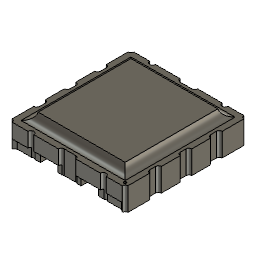
MGF0918A (Autodesk Fusion 360 design; units mm, degrees)
part number: 2026-08-04-15-31-29-317
Autodesk Fusion 360 part; units mm, degrees
sketch "Sketch1" plane through (0, 0, 0) normal (0, 0, 1) x (1, 0, 0)
  line L0 (2, 2.1) -> (-2, 2.1)
  line L1 (-2, 2.1) -> (-2, -2.1)
  line L2 (-2, -2.1) -> (2, -2.1)
  line L3 (2, -2.1) -> (2, 2.1)
  line L4 (2, 2.1) -> (-2, -2.1) construction
  line L5 (-2, 2.1) -> (2, -2.1) construction
  dimension "d1" = 4
  dimension "d2" = 4.2
  constraint horizontal L0
  constraint perpendicular L0 L1
  constraint parallel L0 L2
  constraint parallel L1 L3
  constraint coincident L4 origin
  constraint coincident L5 origin
  measures "d1" distance of L1.end L2.end
  measures "d2" distance of L0.end L1.end
extrude "Extrude1" add sketch "Sketch1" along normal blind 0.8
sketch "Sketch2" plane through (0, 0, 0.8) normal (0, 0, 1) x (-1, 0, 0)
  line L0 (-2, 2.1) -> (-2, -2.1)
  line L1 (-2, -2.1) -> (2, -2.1)
  line L2 (2, -2.1) -> (2, 2.1)
  line L3 (2, 2.1) -> (-2, 2.1)
sketch "Sketch3" plane through (0, 0, 0.8) normal (0, 0, 1) x (-1, 0, 0)
  line L0 (-2, -2.1) -> (2, -2.1)
  line L1 (-1.5, -1.6) -> (1.5, -1.6)
  line L2 (1.5, -1.6) -> (1.5, 1.6)
  line L3 (1.5, 1.6) -> (-1.5, 1.6)
  line L4 (-1.5, 1.6) -> (-1.5, -1.6)
  line L5 (-1.5, -1.6) -> (1.5, 1.6) construction
  line L6 (1.5, -1.6) -> (-1.5, 1.6) construction
  dimension "d5" = 4
  dimension "d6" = 3
  dimension "d7" = 3.2
  constraint horizontal L1
  constraint perpendicular L1 L2
  constraint parallel L1 L3
  constraint parallel L2 L4
  constraint coincident L5 origin
  constraint coincident L6 origin
  measures "d5" distance of L0.start L0.end
  measures "d6" distance of L2.end L3.end
  measures "d7" distance of L1.end L2.end
extrude "Extrude2" add sketch "Sketch3" along normal blind 0.25
sketch "Sketch4" plane through (0, 0, 0) normal (0, 0, -1) x (1, 0, 0)
  line L0 (2, -2.1) -> (2, 2.1)
  line L1 (2, 2.1) -> (-2, 2.1)
  line L2 (-2, 2.1) -> (-2, -2.1)
  line L3 (-2, -2.1) -> (2, -2.1)
  line L4 (-2, -2.1) -> (2, -2.1) construction
  line L5 (0, -2.1) -> (0, -2) construction
  line L6 (0.3, -2.1) -> (0.3, -2) construction
  line L7 (-0.3, -2.1) -> (-0.3, -2) construction
  line L8 (1.25, -2.1) -> (1.25, -2) construction
  line L9 (-1.25, -2.1) -> (-1.25, -2) construction
  line L10 (1.35, -2.1) -> (1.35, -2) construction
  line L11 (1.15, -2.1) -> (1.15, -2) construction
  line L12 (1.35, -2.1) -> (1.15, -2.1)
  arc A0 (1.25, -2) -> (1.15, -2.1) centre (1.25, -2.1) ccw
  arc A1 (1.35, -2.1) -> (1.25, -2) centre (1.25, -2.1) ccw
  arc A2 (-1.25, -2) -> (-1.35, -2.1) centre (-1.25, -2.1) ccw
  arc A3 (-1.15, -2.1) -> (-1.25, -2) centre (-1.25, -2.1) ccw
  line L13 (-1.15, -2.1) -> (-1.35, -2.1)
  line L14 (-0.2, -2) -> (0.2, -2)
  line L15 (0.3, -2.1) -> (-0.3, -2.1)
  arc A4 (-0.2, -2) -> (-0.3, -2.1) centre (-0.2, -2.1) ccw
  arc A5 (0.3, -2.1) -> (0.2, -2) centre (0.2, -2.1) ccw
  arc A6 (1.15, 2.1) -> (1.25, 2) centre (1.25, 2.1) ccw
  arc A7 (1.25, 2) -> (1.35, 2.1) centre (1.25, 2.1) ccw
  line L16 (-0.2, 2) -> (0.2, 2)
  arc A8 (-0.3, 2.1) -> (-0.2, 2) centre (-0.2, 2.1) ccw
  arc A9 (0.2, 2) -> (0.3, 2.1) centre (0.2, 2.1) ccw
  arc A10 (-1.35, 2.1) -> (-1.25, 2) centre (-1.25, 2.1) ccw
  arc A11 (-1.25, 2) -> (-1.15, 2.1) centre (-1.25, 2.1) ccw
  line L17 (1.35, 2.1) -> (1.15, 2.1)
  line L18 (-0.3, 2.1) -> (0.3, 2.1)
  line L19 (-1.15, 2.1) -> (-1.35, 2.1)
  line L20 (0, 0) -> (2, 0) construction
  line L21 (0, 0) -> (-2, 0) construction
  line L22 (2, 0) -> (2, 0.2)
  line L23 (2, 0) -> (2, -0.2)
  line L24 (1.9, 0.1) -> (1.9, -0.1)
  arc A12 (2, 0.2) -> (1.9, 0.1) centre (2, 0.1) ccw
  arc A13 (1.9, -0.1) -> (2, -0.2) centre (2, -0.1) ccw
  arc A14 (-2, -0.2) -> (-1.9, -0.1) centre (-2, -0.1) ccw
  line L25 (-2, 0) -> (-2, -0.2)
  line L26 (-2, 0) -> (-2, 0.2)
  arc A15 (-1.9, 0.1) -> (-2, 0.2) centre (-2, 0.1) ccw
  line L27 (-1.9, 0.1) -> (-1.9, -0.1)
  arc A16 (1.9, 0.95) -> (2, 0.85) centre (2, 0.95) ccw
  line L28 (2, 1.05) -> (2, 0.85)
  line L29 (2, 1.05) -> (2, 1.25)
  arc A17 (2, 1.25) -> (1.9, 1.15) centre (2, 1.15) ccw
  line L30 (1.9, 1.15) -> (1.9, 0.95)
  arc A18 (1.9, -1.15) -> (2, -1.25) centre (2, -1.15) ccw
  line L31 (2, -1.05) -> (2, -1.25)
  line L32 (2, -1.05) -> (2, -0.85)
  arc A19 (2, -0.85) -> (1.9, -0.95) centre (2, -0.95) ccw
  line L33 (1.9, -0.95) -> (1.9, -1.15)
  arc A20 (-2, 0.85) -> (-1.9, 0.95) centre (-2, 0.95) ccw
  line L34 (-2, 1.05) -> (-2, 0.85)
  line L35 (-2, 1.05) -> (-2, 1.25)
  line L36 (-1.9, 1.15) -> (-1.9, 0.95)
  arc A21 (-1.9, 1.15) -> (-2, 1.25) centre (-2, 1.15) ccw
  arc A22 (-2, -1.25) -> (-1.9, -1.15) centre (-2, -1.15) ccw
  line L37 (-2, -1.05) -> (-2, -1.25)
  line L38 (-2, -1.05) -> (-2, -0.85)
  line L39 (-1.9, -0.95) -> (-1.9, -1.15)
  arc A23 (-1.9, -0.95) -> (-2, -0.85) centre (-2, -0.95) ccw
  line L40 (-2, 2.1) -> (-2, 2)
  line L41 (-2, 2.1) -> (-1.9, 2.1)
  arc A24 (-2, 2) -> (-1.9, 2.1) centre (-2.0025, 2.1025) ccw
  line L42 (5.9981, 2.0992) -> (6.0981, 2.0992)
  line L43 (5.9981, 2.0992) -> (5.9981, 1.9992)
  arc A25 (5.9981, 1.9992) -> (6.0981, 2.0992) centre (5.9956, 2.1017) ccw
  line L44 (2, 2.1) -> (1.9, 2.1)
  line L45 (2, 2.1) -> (2, 2)
  arc A26 (1.9, 2.1) -> (2, 2) centre (2.0025, 2.1025) ccw
  arc A27 (2, -2) -> (1.9, -2.1) centre (2.0025, -2.1025) ccw
  line L46 (2, -2.1) -> (2, -2)
  line L47 (2, -2.1) -> (1.9, -2.1)
  line L48 (-2, -2.1) -> (-2, -2)
  line L49 (-2, -2.1) -> (-1.9, -2.1)
  arc A28 (-1.9, -2.1) -> (-2, -2) centre (-2.0025, -2.1025) ccw
  point P0 (0, -2.1)
  constraint coincident L0.start L3.end
  constraint midpoint L3 P0
  constraint coincident P0 L5.start
  constraint perpendicular L4 L5
  constraint horizontal L12
  constraint coincident L11.start L12.end
  constraint coincident L8.end A0.start
  constraint coincident L10.start L12.start
  constraint horizontal L13
  constraint coincident A2.end L13.end
  constraint coincident L9.end A2.start
  constraint coincident A3.start L13.start
  constraint horizontal L14
  constraint horizontal L15
  constraint coincident L7.end L14
  constraint tangent L14 A4
  constraint coincident L7.start L15.end
  constraint tangent L14 A5
  constraint coincident L6.start L15.start
  constraint parallel L1 L17
  constraint parallel L1 L18
  constraint parallel L1 L19
  constraint coincident L20.start L21.start
  constraint midpoint L2 L21.end
  constraint coincident L0 L22.end
  constraint perpendicular L20 L22
  constraint coincident L0 L23.end
  constraint perpendicular L20 L23
  constraint perpendicular L20 L24
  constraint coincident L22.end A12.start
  constraint tangent L24 A13
  constraint coincident L23.end A13.end
  constraint coincident L29.end A17.start
  constraint tangent A16 L30
  constraint coincident A16.end L28.end
  constraint coincident L32.end A19.start
  constraint tangent A18 L33
  constraint coincident A18.end L31.end
  constraint coincident L1.end L2.start
  constraint coincident L2 L40.end
  constraint coincident L1 L41.end
extrude "Extrude3" cut sketch "Sketch4" against normal blind 0.8 contours L0 A18 L31 L32 A19 L33 | L3 L12 A0 A1 | L3 L14 L15 A4 A5 | L0 L22 L23 L24 A12 A13 | L3 A2 A3 L13 | L0 A16 L28 L29 A17 L30 | L2 A22 L37 L38 L39 A23 | L1 A6 A7 L17 | L2 A14 L25 L26 A15 L27 | L1 L16 A8 A9 L18 | L2 A20 L34 L35 L36 A21 | L1 A10 A11 L19
extrude "Extrude4" cut sketch "Sketch4" against normal blind 0.8 contours L0 L3 A27 L46 L47 | L2 L3 L48 L49 A28 | L0 L1 L44 L45 A26 | L1 L2 L40 L41 A24
sketch "Sketch6" plane through (0, 0, 0) normal (0, 0, -1) x (1, 0, 0)
  arc A0 (2, -2) -> (1.9, -2.1) centre (2.0025, -2.1025) ccw
  line L0 (2, -2) -> (2, -1.25)
  arc A1 (1.9, -1.15) -> (2, -1.25) centre (2, -1.15) ccw
  line L1 (1.9, -1.15) -> (1.9, -0.95)
  arc A2 (2, -0.85) -> (1.9, -0.95) centre (2, -0.95) ccw
  line L2 (2, -0.85) -> (2, -0.2)
  arc A3 (1.9, -0.1) -> (2, -0.2) centre (2, -0.1) ccw
  line L3 (1.9, -0.1) -> (1.9, 0.1)
  arc A4 (2, 0.2) -> (1.9, 0.1) centre (2, 0.1) ccw
  line L4 (2, 0.2) -> (2, 0.85)
  arc A5 (1.9, 0.95) -> (2, 0.85) centre (2, 0.95) ccw
  line L5 (1.9, 0.95) -> (1.9, 1.15)
  arc A6 (2, 1.25) -> (1.9, 1.15) centre (2, 1.15) ccw
  line L6 (2, 1.25) -> (2, 2)
  arc A7 (1.9, 2.1) -> (2, 2) centre (2.0025, 2.1025) ccw
  line L7 (1.9, 2.1) -> (1.35, 2.1)
  arc A8 (1.15, 2.1) -> (1.35, 2.1) centre (1.25, 2.1) ccw
  line L8 (1.15, 2.1) -> (0.3, 2.1)
  arc A9 (0.2, 2) -> (0.3, 2.1) centre (0.2, 2.1) ccw
  line L9 (0.2, 2) -> (-0.2, 2)
  arc A10 (-0.3, 2.1) -> (-0.2, 2) centre (-0.2, 2.1) ccw
  line L10 (-0.3, 2.1) -> (-1.15, 2.1)
  arc A11 (-1.35, 2.1) -> (-1.15, 2.1) centre (-1.25, 2.1) ccw
  line L11 (-1.35, 2.1) -> (-1.9, 2.1)
  arc A12 (-2, 2) -> (-1.9, 2.1) centre (-2.0025, 2.1025) ccw
  line L12 (-2, 2) -> (-2, 1.25)
  arc A13 (-1.9, 1.15) -> (-2, 1.25) centre (-2, 1.15) ccw
  line L13 (-1.9, 1.15) -> (-1.9, 0.95)
  arc A14 (-2, 0.85) -> (-1.9, 0.95) centre (-2, 0.95) ccw
  line L14 (-2, 0.85) -> (-2, 0.2)
  arc A15 (-1.9, 0.1) -> (-2, 0.2) centre (-2, 0.1) ccw
  line L15 (-1.9, 0.1) -> (-1.9, -0.1)
  arc A16 (-2, -0.2) -> (-1.9, -0.1) centre (-2, -0.1) ccw
  line L16 (-2, -0.2) -> (-2, -0.85)
  arc A17 (-1.9, -0.95) -> (-2, -0.85) centre (-2, -0.95) ccw
  line L17 (-1.9, -0.95) -> (-1.9, -1.15)
  arc A18 (-2, -1.25) -> (-1.9, -1.15) centre (-2, -1.15) ccw
  line L18 (-2, -1.25) -> (-2, -2)
  arc A19 (-1.9, -2.1) -> (-2, -2) centre (-2.0025, -2.1025) ccw
  line L19 (-1.9, -2.1) -> (-1.35, -2.1)
  arc A20 (-1.15, -2.1) -> (-1.35, -2.1) centre (-1.25, -2.1) ccw
  line L20 (-1.15, -2.1) -> (-0.3, -2.1)
  arc A21 (-0.2, -2) -> (-0.3, -2.1) centre (-0.2, -2.1) ccw
  line L21 (-0.2, -2) -> (0.2, -2)
  arc A22 (0.3, -2.1) -> (0.2, -2) centre (0.2, -2.1) ccw
  line L22 (0.3, -2.1) -> (1.15, -2.1)
  arc A23 (1.35, -2.1) -> (1.15, -2.1) centre (1.25, -2.1) ccw
  line L23 (1.35, -2.1) -> (1.9, -2.1)
  line L24 (0, 0) -> (0, -0.6) construction
  line L25 (0, -0.6) -> (1, -0.6)
  line L26 (1, -0.6) -> (1, -2.0203)
  line L27 (1, -2.0203) -> (1.8, -2.0203)
  line L28 (1.8, -2.0203) -> (1.9, -2.1)
  line L29 (0, -0.6) -> (-1, -0.6)
  line L30 (-1, -0.6) -> (-1, -2.0203)
  line L31 (-1, -2.0203) -> (-1.8, -2.0203)
  line L32 (-1.8, -2.0203) -> (-1.9, -2.1)
  line L33 (1, -2.0203) -> (-1, -2.0203) construction
  line L34 (0, -2.0203) -> (0.4, -2.0203)
  line L35 (0, -2.0203) -> (-0.4, -2.0203)
  line L36 (-0.4, -2.0203) -> (-0.4, -1.3203)
  line L37 (-0.4, -1.3203) -> (0.4, -1.3203)
  line L38 (0.4, -1.3203) -> (0.4, -2.0203)
  line L39 (1.9, 0) -> (-1.9, 0) construction
  line L40 (0, 2.0203) -> (0.4, 2.0203)
  line L41 (0, 2.0203) -> (-0.4, 2.0203)
  line L42 (-0.4, 2.0203) -> (-0.4, 1.3203)
  line L43 (-0.4, 1.3203) -> (0.4, 1.3203)
  line L44 (0.4, 1.3203) -> (0.4, 2.0203)
  line L45 (0, 2.1) -> (0, 0.6) construction
  line L46 (0, 0.6) -> (1, 0.6)
  line L47 (1, 2.0203) -> (1.8, 2.0203)
  line L48 (1.8, 2.0203) -> (1.9, 2.1)
  line L49 (-1, 2.0203) -> (-1.8, 2.0203)
  line L50 (-1.8, 2.0203) -> (-1.9, 2.1)
  line L51 (0, 0.6) -> (-1, 0.6)
  line L52 (1.25, 2) -> (1.25, 0.6) construction
  line L53 (1, 0.6) -> (1.25, 0.6)
  line L54 (1.25, 0.6) -> (1.25, 0.85)
  line L55 (1.25, 0.85) -> (1, 0.85)
  line L56 (1, 0.85) -> (1, 2.0203)
  line L57 (-1, 0.85) -> (-1, 2.0203)
  line L58 (-1.25, 0.85) -> (-1, 0.85)
  line L59 (-1.25, 0.6) -> (-1.25, 0.85)
  line L60 (-1.25, 0.6) -> (-1, 0.6)
  line L61 (-1.9, 2.1) -> (1.9, 2.1)
  line L62 (1.9, -2.1) -> (-1.9, -2.1)
  dimension "d38" = 0.7
  dimension "d39" = 0.6
  dimension "d40" = 0.6
  constraint coincident L24.start origin
  constraint perpendicular L8 L24
  constraint perpendicular L24 L25
  constraint perpendicular L22 L26
  constraint perpendicular L26 L27
  constraint coincident A0.end L23.end
  constraint symmetric L25.start L24 L29.start
  constraint symmetric L24 L25.end L29.end
  constraint symmetric L24 L26.end L30.end
  constraint symmetric L24 L27.end L31.end
  constraint symmetric L24 A0.end A19.start
  constraint midpoint L33 L34.start
  constraint coincident L33 L34.end
  constraint coincident L33 L35.end
  constraint perpendicular L35 L36
  constraint perpendicular L36 L37
  constraint perpendicular L33 L38
  constraint midpoint L3 L39.start
  constraint midpoint L15 L39.end
  constraint symmetric L34.start L39 L40.start
  constraint symmetric L34.end L39 L40.end
  constraint symmetric L35.end L39 L41.end
  constraint symmetric L36.end L39 L42.end
  constraint symmetric L37.end L39 L43.end
  constraint perpendicular L41 L45
  constraint symmetric L24.end L39 L45.end
  constraint symmetric L25.end L39 L46.end
  constraint symmetric L26.end L39 L47.start
  constraint symmetric L27.end L39 L47.end
  constraint symmetric A0.end L39 A7.start
  constraint symmetric L29.end L39 L51.end
  constraint symmetric L30.end L39 L49.start
  constraint symmetric L31.end L39 L49.end
  constraint symmetric A19.start L39 L11.end
  constraint midpoint A8 L52.start
  constraint perpendicular L47 L52
  constraint perpendicular L52 L53
  constraint coincident L52 L54.end
  constraint perpendicular L47 L56
  constraint symmetric L45 L47.start L49.start
  constraint symmetric L45 L52.end L59.start
  constraint symmetric L45 L54.end L58.start
  constraint symmetric L45 L55.end L57.start
  constraint perpendicular L59 L60
  measures "d38" distance of L35.end L36.end
  measures "d39" distance of L25.end L39
  measures "d40" distance of L24.start L45.end
extrude "Extrude5" cut sketch "Sketch6" against normal blind 0.3 contours A23 L23 L27 L28 L62 | A20 L20 A21 A22 L22 A23 L25 L26 L27 L29 L30 L31 L34 L35 L36 L37 L38 L62 | L19 A20 L31 L32 L62 | L7 A8 L47 L48 L61 | A8 L8 A9 A10 L10 A11 L40 L41 L42 L43 L44 L46 L47 L49 L51 L53 L54 L55 L56 L57 L58 L59 L60 L61 | A11 L11 L49 L50 L61
fillet "Fillet1" radius 0.3 1 edges at (0, 1.6, 0.8)
fillet "Fillet2" radius 0.3 1 edges at (-1.5, 0.1479, 0.8)
fillet "Fillet3" radius 0.3 2 edges at (-0.1479, -1.6, 0.8) (1.5, 0.1479, 0.8)
sketch "Sketch7" plane through (0, 0, 0.8) normal (0, 0, 1) x (-1, 0, 0)
  arc A0 (-1.9, -2.1) -> (-2, -2) centre (-2.0025, -2.1025) ccw
  line L0 (-1.9, -2.1) -> (-1.35, -2.1)
  arc A1 (-1.15, -2.1) -> (-1.35, -2.1) centre (-1.25, -2.1) ccw
  line L1 (-1.15, -2.1) -> (-0.3, -2.1)
  arc A2 (-0.2, -2) -> (-0.3, -2.1) centre (-0.2, -2.1) ccw
  line L2 (-0.2, -2) -> (0.2, -2)
  arc A3 (0.3, -2.1) -> (0.2, -2) centre (0.2, -2.1) ccw
  line L3 (0.3, -2.1) -> (1.15, -2.1)
  arc A4 (1.35, -2.1) -> (1.15, -2.1) centre (1.25, -2.1) ccw
  line L4 (1.35, -2.1) -> (1.9, -2.1)
  arc A5 (2, -2) -> (1.9, -2.1) centre (2.0025, -2.1025) ccw
  line L5 (2, -2) -> (2, -1.25)
  arc A6 (1.9, -1.15) -> (2, -1.25) centre (2, -1.15) ccw
  line L6 (1.9, -1.15) -> (1.9, -0.95)
  arc A7 (2, -0.85) -> (1.9, -0.95) centre (2, -0.95) ccw
  line L7 (2, -0.85) -> (2, -0.2)
  arc A8 (1.9, -0.1) -> (2, -0.2) centre (2, -0.1) ccw
  line L8 (1.9, -0.1) -> (1.9, 0.1)
  arc A9 (2, 0.2) -> (1.9, 0.1) centre (2, 0.1) ccw
  line L9 (2, 0.2) -> (2, 0.85)
  arc A10 (1.9, 0.95) -> (2, 0.85) centre (2, 0.95) ccw
  line L10 (1.9, 0.95) -> (1.9, 1.15)
  arc A11 (2, 1.25) -> (1.9, 1.15) centre (2, 1.15) ccw
  line L11 (2, 1.25) -> (2, 2)
  arc A12 (1.9, 2.1) -> (2, 2) centre (2.0025, 2.1025) ccw
  line L12 (1.9, 2.1) -> (1.35, 2.1)
  arc A13 (1.15, 2.1) -> (1.35, 2.1) centre (1.25, 2.1) ccw
  line L13 (1.15, 2.1) -> (0.3, 2.1)
  arc A14 (0.2, 2) -> (0.3, 2.1) centre (0.2, 2.1) ccw
  line L14 (0.2, 2) -> (-0.2, 2)
  arc A15 (-0.3, 2.1) -> (-0.2, 2) centre (-0.2, 2.1) ccw
  line L15 (-0.3, 2.1) -> (-1.15, 2.1)
  arc A16 (-1.35, 2.1) -> (-1.15, 2.1) centre (-1.25, 2.1) ccw
  line L16 (-1.35, 2.1) -> (-1.9, 2.1)
  arc A17 (-2, 2) -> (-1.9, 2.1) centre (-2.0025, 2.1025) ccw
  line L17 (-2, 2) -> (-2, 1.25)
  arc A18 (-1.9, 1.15) -> (-2, 1.25) centre (-2, 1.15) ccw
  line L18 (-1.9, 1.15) -> (-1.9, 0.95)
  arc A19 (-2, 0.85) -> (-1.9, 0.95) centre (-2, 0.95) ccw
  line L19 (-2, 0.85) -> (-2, 0.2)
  arc A20 (-1.9, 0.1) -> (-2, 0.2) centre (-2, 0.1) ccw
  line L20 (-1.9, 0.1) -> (-1.9, -0.1)
  arc A21 (-2, -0.2) -> (-1.9, -0.1) centre (-2, -0.1) ccw
  line L21 (-2, -0.2) -> (-2, -0.85)
  arc A22 (-1.9, -0.95) -> (-2, -0.85) centre (-2, -0.95) ccw
  line L22 (-1.9, -0.95) -> (-1.9, -1.15)
  arc A23 (-2, -1.25) -> (-1.9, -1.15) centre (-2, -1.15) ccw
  line L23 (-2, -1.25) -> (-2, -2)
  line L24 (1.7958, -1.8958) -> (-1.7958, -1.8958)
  line L25 (-1.7958, -1.8958) -> (-1.7958, 1.8958)
  line L26 (-1.7958, 1.8958) -> (1.7958, 1.8958)
  line L27 (1.7958, 1.8958) -> (1.7958, -1.8958)
  circle A24 centre (-1.85, 1.95) radius 0.04
extrude "Extrude6" cut sketch "Sketch7" against normal blind 0.01 contours A24
